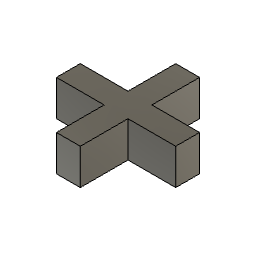
piece v2 (Autodesk Fusion 360 design; units mm, degrees)
Autodesk Fusion 360 part; units mm, degrees
sketch "Sketch1" plane through (0, 0, 0) normal (0, 0, 1) x (1, 0, 0)
  line L0 (0, 0) -> (10, 0)
  line L1 (10, 0) -> (10, 50)
  line L2 (10, 50) -> (0, 50)
  line L3 (0, 50) -> (0, 0)
  line L4 (0, 0) -> (0, 20) construction
  line L5 (0, 50) -> (0, 30) construction
  line L6 (0, 20) -> (-20, 20)
  line L7 (-20, 20) -> (-20, 30)
  line L8 (-20, 30) -> (0, 30)
  line L9 (0, 30) -> (0, 20)
  line L10 (0, 30) -> (10, 30) construction
  line L11 (10, 30) -> (30, 30)
  line L12 (30, 30) -> (30, 20)
  line L13 (30, 20) -> (10, 20)
  line L14 (10, 20) -> (10, 30)
  dimension "d1" = 10
  dimension "d2" = 50
  dimension "d3" = 20
  dimension "d4" = 20
  dimension "d5" = 20
  dimension "d6" = 10
  dimension "d7" = 20
  dimension "d8" = 10
  constraint horizontal L0
  constraint vertical L1
  constraint horizontal L2
  constraint vertical L3
  constraint coincident L0.start L3.end
  constraint perpendicular L0 L4
  constraint perpendicular L2 L5
  constraint horizontal L6
  constraint vertical L7
  constraint horizontal L8
  constraint vertical L9
  constraint coincident L1 L10.end
  constraint perpendicular L1 L10
  constraint horizontal L11
  constraint vertical L12
  constraint horizontal L13
  constraint vertical L14
  measures "d1" distance of L0.start L0.end
  measures "d2" distance of L0.start L2.end
  measures "d3" distance of L0.start L4.end
  measures "d4" distance of L2.end L5.end
  measures "d5" distance of L4.end L6.end
  measures "d6" distance of L4.end L5.end
  measures "d7" distance of L10.end L11.end
  measures "d8" distance of L10.end L13.end
extrude "Extrude1" add sketch "Sketch1" along normal blind 15
sketch "Sketch2" plane through (0, 0, 0) normal (0, 0, -1) x (1, 0, 0)
  line L0 (10, -50) -> (10, -30)
  line L1 (10, -30) -> (30, -30)
  line L2 (30, -30) -> (30, -20)
  line L3 (30, -20) -> (10, -20)
  line L4 (10, -20) -> (10, 0)
  line L5 (10, 0) -> (0, 0)
  line L6 (0, 0) -> (0, -20)
  line L7 (0, -20) -> (-20, -20)
  line L8 (-20, -20) -> (-20, -30)
  line L9 (-20, -30) -> (0, -30)
  line L10 (0, -30) -> (0, -50)
  line L11 (0, -50) -> (10, -50)
  line L12 (5, 0) -> (5, -3) construction
  circle A0 centre (5, -3) radius 2.25
  dimension "d11" = 3
  dimension "d12" = 4.5
  constraint midpoint L5 L12.start
  constraint perpendicular L5 L12
  constraint coincident L12.end A0.centre
  measures "d11" distance of L12.start L12.end
  measures "d12" diameter of A0
sketch "Sketch3" plane through (0, 0, 0) normal (-1, 0, 0) x (0, -1, 0)
  line L0 (-20, 0) -> (0, 0)
  line L1 (0, 0) -> (0, 15)
  line L2 (0, 15) -> (-20, 15)
  line L3 (-20, 15) -> (-20, 0)
  spline S0 degree 5 poles (-2.1325, 0) (-2.2809, 0.367) (-2.5879, 1.0837) (-3.0793, 2.107) (-3.7967, 3.3673) (-4.7984, 4.7664) (-5.9064, 5.9851) (-7.1214, 7.0186) (-8.4425, 7.862) (-9.8666, 8.5117) (-11.3865, 8.9649) (-12.9891, 9.2196) (-14.6534, 9.275) (-16.3483, 9.1317) (-18.0298, 8.7919) (-19.6458, 8.2591) (-21.1423, 7.5377) (-22.469, 6.6324) (-23.5849, 5.5483) (-24.4652, 4.2906) (-25.0983, 2.8644) (-25.4042, 1.5919) (-25.5213, 0.5648) (-25.5496, -0.1522) (-25.5513, -0.5187) knots 0 0 0 0 0 0 0.05 0.1 0.15 0.2 0.25 0.3 0.35 0.4 0.45 0.5 0.55 0.6 0.65 0.7 0.75 0.8 0.85 0.9 0.95 1 1 1 1 1 1
  point P0 (-7.4581, 7.1927)
  point P1 (-14.864, 9.2186)
  point P2 (-22.6118, 6.4236)
sweep "Sweep1" cut profiles "Sketch2" path "Sketch3" along S0 section 1 contours A0
